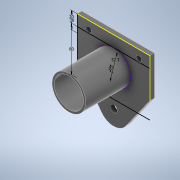
# Autodesk Inventor part: encaje
Saved by Autodesk Inventor 2021 (Build 250183000, 183)
## iProperties
Created: 2022-01-26
Part Number: encaje
Material: Genérico
Document SubType Name: Modeling
Designer: arthu
Density: 1 g/cm^3
Appearance: Suave - Negro
Author: arthu
Autodesk Inventor part; units mm, degrees
ref_plane "YZ Plane" through (0, 0, 0) normal (1, 0, 0) x (0, 1, 0)
ref_plane "XZ Plane" through (0, 0, 0) normal (0, 1, 0) x (-1, 0, 0)
ref_plane "XY Plane" through (0, 0, 0) normal (0, 0, 1) x (1, 0, 0)
sketch "Boceto1" plane through (0, 0, 0) normal (0, 0, 1) x (1, 0, 0)
  line L0 (0, 0) -> (0, 40)
  line L1 (65, 70) -> (-65, 70)
  line L2 (-65, 70) -> (-65, 10)
  line L3 (-65, 10) -> (65, 10)
  line L4 (65, 10) -> (65, 70)
  line L5 (65, 70) -> (-65, 10) construction
  line L6 (-65, 70) -> (65, 10) construction
  line L7 (65, 70) -> (-65, 70)
  line L8 (-65, 70) -> (-65, 0)
  line L9 (65, 0) -> (65, 70)
  line L10 (65, 70) -> (65, 40)
  line L11 (65, 55) -> (-65, 55)
  line L12 (65, 55) -> (45, 55)
  circle A0 centre (45, 55) radius 5
  line L13 (-65, 55) -> (-62.9791, 55)
  line L14 (-65, 55) -> (-45, 55)
  circle A1 centre (-45, 55) radius 5
  line L15 (6.5, -45) -> (-6.5, -45)
  circle A2 centre (0, -45) radius 6.5
  arc A3 (-22.0262, -60.6156) -> (22.0262, -60.6156) centre (0, -45) ccw
  line L16 (65, 0) -> (22.0262, -60.6156)
  line L17 (-65, 0) -> (-22.0262, -60.6156)
  dimension "d0" = 130
  dimension "d1" = 60
  dimension "d2" = 20
  dimension "d3" = 10
  dimension "d4" = 20
  dimension "d5" = 10
  dimension "d6" = 13
  constraints: 36 end point, 5 point on line, 4 centre point, 4 midpoint, 4 perpendicular, 4 point on circle, 3 coincident, 3 parallel, 2 horizontal, 2 tangent
  measures "d0" distance of L4.start L2.end
  measures "d1" distance of L2.end L2.start
  measures "d2" distance of L12.start L12.end
  measures "d3" diameter of A0
  measures "d4" distance of L13.start L14.end
  measures "d5" diameter of A1
  measures "d6" diameter of A2
extrude "Extrusión1" add sketch "Boceto1" along normal blind 8 contours L4 L11 A0 A1 L2 L1 | L4 L3 L2 L11 A1 A0 | L3 L9 L16 A3 L17 L8
sketch "Boceto2" plane through (0, 0, 8) normal (0, 0, 1) x (1, 0, 0)
  line L0 (65, 70) -> (-65, 70) projected
  line L1 (-65, 70) -> (-65, 40)
  line L2 (-65, 70) -> (-65, 0) projected
  line L3 (65, 0) -> (65, 70) projected
  line L4 (-65, 70) -> (-65, 50)
  line L5 (-65, 50) -> (65, 50)
  line L6 (-65, 50) -> (-65, -30)
  line L7 (-65, -30) -> (65, -30)
  line L8 (0, 50) -> (0, -30)
  line L9 (0, 10) -> (0, 20)
  circle A0 centre (0, 20) radius 30
  circle A1 centre (0, 20) radius 26.15
  point P0 (0, 0)
  dimension "d13" = 30
  dimension "d15" = 20
  dimension "d16" = 80
  dimension "d23" = 10
  dimension "d24" = 52.3
  constraints: 14 end point, 5 point on line, 3 midpoint, 2 coincident, 2 perpendicular, 1 centre point, 1 vertical alignment, 2 other
  measures "d13" distance of L0.end L1.end
  measures "d15" distance of L0.end L4.end
  measures "d16" distance of L4.end L6.end
  measures "d23" distance of L9.start L9.end
  measures "d24" diameter of A1
extrude "Extrusión4" add sketch "Boceto2" along normal blind 80 contours A0 L8 A1 | L8 A1 A0
